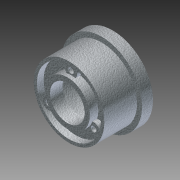
# Autodesk Inventor part: Drill Dap 1.6925 D Dewalt XRP
Saved by Autodesk Inventor 2012 (Build 160160000, 160)
## iProperties
Created: 2012-07-04
Part Number: Drill Dap 1.6925 D Dewalt XRP
Material: Default
Document SubType Name: Modeling
Designer: Bruce
Density: 1 g/cm^3
Author: Bruce
Autodesk Inventor part; units mm, degrees
ref_plane "YZ Plane" through (0, 0, 0) normal (1, 0, 0) x (0, 1, 0)
ref_plane "XZ Plane" through (0, 0, 0) normal (0, 1, 0) x (-1, 0, 0)
ref_plane "XY Plane" through (0, 0, 0) normal (0, 0, 1) x (1, 0, 0)
sketch "Sketch1" plane through (0, 0, 0) normal (0, 0, 1) x (1, 0, 0)
  circle A0 centre (0, 0) radius 24.4793
  circle A1 centre (0, 0) radius 21.4312
  circle A2 centre (0, 0) radius 19.5263
  circle A3 centre (0, 0) radius 13.6017
  circle A4 centre (0, 0) radius 10.5093
  dimension "d0" = 48.9585
  dimension "d1" = 42.8625
  dimension "d2" = 39.0525
  dimension "d3" = 27.2034
  dimension "d4" = 21.0185
  constraints: 5 centre point, 5 coincident
  measures "d0" diameter of A0
  measures "d1" diameter of A1
  measures "d2" diameter of A2
  measures "d3" diameter of A3
  measures "d4" diameter of A4
extrude "Extrusion1" add sketch "Sketch1" against normal blind 27.4955 contours A0 | A1 | A2 | A3
extrude "Extrusion2" cut sketch "Sketch1" against normal blind 20.8534 contours A0
extrude "Extrusion3" cut sketch "Sketch1" against normal blind 5.1562 contours A2
extrude "Extrusion4" cut sketch "Sketch1" against normal blind 1.016 contours A1
sketch "Sketch2" plane through (0, 0, -5.1562) normal (0, 0, 1) x (1, 0, 0)
  circle A0 centre (0, 0) radius 13.6017 projected
  circle A1 centre (0, 15.875) radius 1.6193
  circle A2 centre (0, 15.875) radius 3.7147
  circle A3 centre (-13.7482, -7.9375) radius 1.6193
  circle A4 centre (-13.7482, -7.9375) radius 3.7147
  circle A5 centre (13.7482, -7.9375) radius 1.6193
  circle A6 centre (13.7482, -7.9375) radius 3.7147
  dimension "d13" = 3.2385
  dimension "d14" = 7.4295
  dimension "d15" = 15.875
  dimension "d18" = 360
  constraints: 6 centre point, 3 coincident, 1 vertical alignment, 13 other
  measures "d13" diameter of A1
  measures "d14" diameter of A2
  measures "d15" distance of A0.centre A1.centre
extrude "Extrusion5" add sketch "Sketch2" along normal blind 2.9337 contours A2 A0 | A0 A2 | A6 A0 | A0 A6 | A4 A0 | A0 A4
sketch "Sketch3" plane through (0, 0, -27.4955) normal (0, 0, -1) x (-1, 0, 0)
  circle A0 centre (0, 0) radius 10.5093 projected
  circle A1 centre (0, 0) radius 24.4793 projected
  circle A2 centre (0, 0) radius 23.114
  circle A3 centre (0, 0) radius 19.4437
  circle A4 centre (0, 0) radius 24.4793
  dimension "d22" = 46.228
  dimension "d23" = 38.8874
  constraints: 3 centre point, 3 coincident, 1 concentric
  measures "d22" diameter of A2
  measures "d23" diameter of A3
extrude "Extrusion6" cut sketch "Sketch3" against normal blind 19.8755 contours A3
extrude "Extrusion7" cut sketch "Sketch3" against normal blind 2.7305 contours A2
extrude "Extrusion8" cut sketch "Sketch2" against normal through all contours A1 | A3 | A5
body "Solid1"
